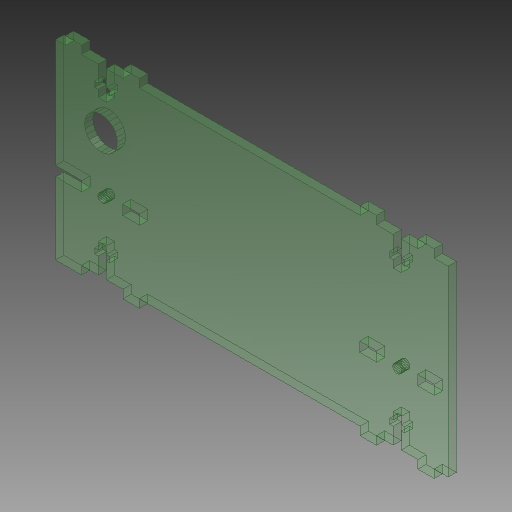
# Autodesk Inventor part: EE-Rear
Saved by Autodesk Inventor 2018 (Build 220112000, 112)
## iProperties
Created: 2016-07-27
Part Number: EE-Rear
Material: Polycarbonate, Green
Document SubType Name: Modeling
Designer: User
Density: 1.2 g/cm^3
Appearance: Polycarbonate - Clear(2)
Author: User
Autodesk Inventor part; units mm, degrees
ref_plane "YZ Plane" through (0, 0, 0) normal (1, 0, 0) x (0, 1, 0)
ref_plane "XZ Plane" through (0, 0, 0) normal (0, 1, 0) x (-1, 0, 0)
ref_plane "XY Plane" through (0, 0, 0) normal (0, 0, 1) x (1, 0, 0)
sketch "Sketch1" plane through (0, 0, 0) normal (0, 0, 1) x (1, 0, 0)
  line L0 (169.4009, -79.2776) -> (169.3009, -79.2776)
  line L1 (169.3009, -79.2776) -> (169.3009, -76.2776)
  line L2 (169.3009, -76.2776) -> (163.3009, -76.2776)
  line L3 (163.3009, -76.2776) -> (163.3009, -79.2776)
  line L4 (163.3009, -79.2776) -> (157.2009, -79.2776)
  line L5 (157.2009, -79.2776) -> (157.2009, -85.2776)
  line L6 (157.2009, -85.2776) -> (158.4509, -85.2776)
  line L7 (158.4509, -85.2776) -> (158.4509, -87.2776)
  line L8 (158.4509, -87.2776) -> (157.2009, -87.2776)
  line L9 (157.2009, -87.2776) -> (157.2009, -89.9276)
  line L10 (157.2009, -89.9276) -> (154.2009, -89.9276)
  line L11 (154.2009, -89.9276) -> (154.2009, -87.2776)
  line L12 (154.2009, -87.2776) -> (152.9509, -87.2776)
  line L13 (152.9509, -87.2776) -> (152.9509, -85.2776)
  line L14 (152.9509, -85.2776) -> (154.2009, -85.2776)
  line L15 (154.2009, -85.2776) -> (154.2009, -79.2776)
  line L16 (154.2009, -79.2776) -> (148.1009, -79.2776)
  line L17 (148.1009, -79.2776) -> (148.1009, -76.2776)
  line L18 (148.1009, -76.2776) -> (142.1009, -76.2776)
  line L19 (142.1009, -76.2776) -> (142.1009, -79.2776)
  line L20 (142.1009, -79.2776) -> (142.0009, -79.2776)
  line L21 (142.0009, -79.2776) -> (61.1009, -79.2776)
  line L22 (61.1009, -79.2776) -> (61.1009, -76.2776)
  line L23 (61.1009, -76.2776) -> (55.1009, -76.2776)
  line L24 (55.1009, -76.2776) -> (55.1009, -79.2776)
  line L25 (55.1009, -79.2776) -> (49.0009, -79.2776)
  line L26 (49.0009, -79.2776) -> (49.0009, -85.2776)
  line L27 (49.0009, -85.2776) -> (50.2509, -85.2776)
  line L28 (50.2509, -85.2776) -> (50.2509, -87.2776)
  line L29 (50.2509, -87.2776) -> (49.0009, -87.2776)
  line L30 (49.0009, -87.2776) -> (49.0009, -89.9276)
  line L31 (49.0009, -89.9276) -> (46.0009, -89.9276)
  line L32 (46.0009, -89.9276) -> (46.0009, -87.2776)
  line L33 (46.0009, -87.2776) -> (44.7509, -87.2776)
  line L34 (44.7509, -87.2776) -> (44.7509, -85.2776)
  line L35 (44.7509, -85.2776) -> (46.0009, -85.2776)
  line L36 (46.0009, -85.2776) -> (46.0009, -79.2776)
  line L37 (46.0009, -79.2776) -> (39.9009, -79.2776)
  line L38 (39.9009, -79.2776) -> (39.9009, -76.2776)
  line L39 (39.9009, -76.2776) -> (34.0009, -76.2776)
  line L40 (34.0009, -76.2776) -> (34.0009, -79.2776)
  line L41 (34.0009, -79.2776) -> (30.4009, -79.2776)
  line L42 (30.4009, -79.2776) -> (30.4009, -119.2776)
  line L43 (30.4009, -119.2776) -> (40.0009, -119.2776)
  line L44 (40.0009, -119.2776) -> (40.0009, -122.8776)
  line L45 (40.0009, -122.8776) -> (30.4009, -122.8776)
  line L46 (30.4009, -122.8776) -> (30.4009, -149.3251)
  line L47 (30.4009, -149.3251) -> (39.901, -149.3251)
  line L48 (39.901, -149.3251) -> (39.901, -146.2776)
  line L49 (39.901, -146.2776) -> (46.0009, -146.2776)
  line L50 (46.0009, -146.2776) -> (46.0009, -140.2776)
  line L51 (46.0009, -140.2776) -> (44.751, -140.2776)
  line L52 (44.751, -140.2776) -> (44.751, -138.2776)
  line L53 (44.751, -138.2776) -> (46.0009, -138.2776)
  line L54 (46.0009, -138.2776) -> (46.0009, -135.6276)
  line L55 (46.0009, -135.6276) -> (49.001, -135.6276)
  line L56 (49.001, -135.6276) -> (49.001, -138.2776)
  line L57 (49.001, -138.2776) -> (50.251, -138.2776)
  line L58 (50.251, -138.2776) -> (50.251, -140.2776)
  line L59 (50.251, -140.2776) -> (49.001, -140.2776)
  line L60 (49.001, -140.2776) -> (49.001, -146.2776)
  line L61 (49.001, -146.2776) -> (55.101, -146.2776)
  line L62 (55.101, -146.2776) -> (55.101, -149.3251)
  line L63 (55.101, -149.3251) -> (61.1009, -149.3251)
  line L64 (61.1009, -149.3251) -> (61.1009, -146.2776)
  line L65 (61.1009, -146.2776) -> (61.2009, -146.2776)
  line L66 (61.2009, -146.2776) -> (142.1009, -146.2776)
  line L67 (142.1009, -146.2776) -> (142.1009, -149.3251)
  line L68 (142.1009, -149.3251) -> (148.1009, -149.3251)
  line L69 (148.1009, -149.3251) -> (148.1009, -146.2776)
  line L70 (148.1009, -146.2776) -> (154.201, -146.2776)
  line L71 (154.201, -146.2776) -> (154.201, -140.2776)
  line L72 (154.201, -140.2776) -> (152.9509, -140.2776)
  line L73 (152.9509, -140.2776) -> (152.9509, -138.2776)
  line L74 (152.9509, -138.2776) -> (154.201, -138.2776)
  line L75 (154.201, -138.2776) -> (154.201, -135.6276)
  line L76 (154.201, -135.6276) -> (157.201, -135.6276)
  line L77 (157.201, -135.6276) -> (157.201, -138.2776)
  line L78 (157.201, -138.2776) -> (158.4509, -138.2776)
  line L79 (158.4509, -138.2776) -> (158.4509, -140.2776)
  line L80 (158.4509, -140.2776) -> (157.201, -140.2776)
  line L81 (157.201, -140.2776) -> (157.201, -146.2776)
  line L82 (157.201, -146.2776) -> (163.3009, -146.2776)
  line L83 (163.3009, -146.2776) -> (163.3009, -149.3251)
  line L84 (163.3009, -149.3251) -> (169.3009, -149.3251)
  line L85 (169.3009, -149.3251) -> (169.3009, -146.2776)
  line L86 (169.3009, -146.2776) -> (169.4009, -146.2776)
  line L87 (169.4009, -146.2776) -> (174.4009, -146.2776)
  line L88 (174.4009, -146.2776) -> (174.4009, -79.2776)
  line L89 (174.4009, -79.2776) -> (169.4009, -79.2776)
  line L90 (52.823, -99.1247) -> (52.2237, -97.6776)
  line L91 (52.2237, -97.6776) -> (51.2701, -96.435)
  line L92 (51.2701, -96.435) -> (50.0275, -95.4815)
  line L93 (50.0275, -95.4815) -> (48.5804, -94.8821)
  line L94 (48.5804, -94.8821) -> (47.0275, -94.6776)
  line L95 (47.0275, -94.6776) -> (45.4746, -94.8821)
  line L96 (45.4746, -94.8821) -> (44.0275, -95.4815)
  line L97 (44.0275, -95.4815) -> (42.7849, -96.435)
  line L98 (42.7849, -96.435) -> (41.8314, -97.6776)
  line L99 (41.8314, -97.6776) -> (41.232, -99.1247)
  line L100 (41.232, -99.1247) -> (41.0275, -100.6776)
  line L101 (41.0275, -100.6776) -> (41.232, -102.2306)
  line L102 (41.232, -102.2306) -> (41.8314, -103.6777)
  line L103 (41.8314, -103.6777) -> (42.7849, -104.9203)
  line L104 (42.7849, -104.9203) -> (44.0275, -105.8738)
  line L105 (44.0275, -105.8738) -> (45.4746, -106.4732)
  line L106 (45.4746, -106.4732) -> (47.0275, -106.6776)
  line L107 (47.0275, -106.6776) -> (48.5804, -106.4732)
  line L108 (48.5804, -106.4732) -> (50.0275, -105.8738)
  line L109 (50.0275, -105.8738) -> (51.2701, -104.9203)
  line L110 (51.2701, -104.9203) -> (52.2237, -103.6777)
  line L111 (52.2237, -103.6777) -> (52.823, -102.2306)
  line L112 (52.823, -102.2306) -> (53.0275, -100.6776)
  line L113 (53.0275, -100.6776) -> (52.823, -99.1247)
  line L114 (49.0226, -120.6837) -> (48.8518, -120.3208)
  line L115 (48.8518, -120.3208) -> (48.5962, -120.0117)
  line L116 (48.5962, -120.0117) -> (48.2718, -119.776)
  line L117 (48.2718, -119.776) -> (47.8988, -119.6284)
  line L118 (47.8988, -119.6284) -> (47.5009, -119.5781)
  line L119 (47.5009, -119.5781) -> (47.103, -119.6284)
  line L120 (47.103, -119.6284) -> (46.7301, -119.776)
  line L121 (46.7301, -119.776) -> (46.4056, -120.0117)
  line L122 (46.4056, -120.0117) -> (46.15, -120.3208)
  line L123 (46.15, -120.3208) -> (45.9792, -120.6837)
  line L124 (45.9792, -120.6837) -> (45.9041, -121.0776)
  line L125 (45.9041, -121.0776) -> (45.9293, -121.4779)
  line L126 (45.9293, -121.4779) -> (46.0532, -121.8594)
  line L127 (46.0532, -121.8594) -> (46.2681, -122.198)
  line L128 (46.2681, -122.198) -> (46.5605, -122.4725)
  line L129 (46.5605, -122.4725) -> (46.9119, -122.6657)
  line L130 (46.9119, -122.6657) -> (47.3004, -122.7655)
  line L131 (47.3004, -122.7655) -> (47.7014, -122.7655)
  line L132 (47.7014, -122.7655) -> (48.09, -122.6657)
  line L133 (48.09, -122.6657) -> (48.4414, -122.4725)
  line L134 (48.4414, -122.4725) -> (48.7337, -122.198)
  line L135 (48.7337, -122.198) -> (48.9486, -121.8594)
  line L136 (48.9486, -121.8594) -> (49.0726, -121.4779)
  line L137 (49.0726, -121.4779) -> (49.0978, -121.0776)
  line L138 (49.0978, -121.0776) -> (49.0226, -120.6837)
  line L139 (142.0009, -119.2776) -> (142.0009, -122.8776)
  line L140 (142.0009, -122.8776) -> (148.2009, -122.8776)
  line L141 (148.2009, -122.8776) -> (148.2009, -119.2776)
  line L142 (148.2009, -119.2776) -> (142.0009, -119.2776)
  line L143 (157.2226, -120.6837) -> (157.0518, -120.3208)
  line L144 (157.0518, -120.3208) -> (156.7962, -120.0117)
  line L145 (156.7962, -120.0117) -> (156.4717, -119.776)
  line L146 (156.4717, -119.776) -> (156.0988, -119.6284)
  line L147 (156.0988, -119.6284) -> (155.7009, -119.5781)
  line L148 (155.7009, -119.5781) -> (155.303, -119.6284)
  line L149 (155.303, -119.6284) -> (154.9301, -119.776)
  line L150 (154.9301, -119.776) -> (154.6056, -120.0117)
  line L151 (154.6056, -120.0117) -> (154.35, -120.3208)
  line L152 (154.35, -120.3208) -> (154.1792, -120.6837)
  line L153 (154.1792, -120.6837) -> (154.1041, -121.0776)
  line L154 (154.1041, -121.0776) -> (154.1292, -121.4779)
  line L155 (154.1292, -121.4779) -> (154.2532, -121.8594)
  line L156 (154.2532, -121.8594) -> (154.4681, -122.198)
  line L157 (154.4681, -122.198) -> (154.7605, -122.4725)
  line L158 (154.7605, -122.4725) -> (155.1119, -122.6657)
  line L159 (155.1119, -122.6657) -> (155.5004, -122.7655)
  line L160 (155.5004, -122.7655) -> (155.9014, -122.7655)
  line L161 (155.9014, -122.7655) -> (156.2899, -122.6657)
  line L162 (156.2899, -122.6657) -> (156.6414, -122.4725)
  line L163 (156.6414, -122.4725) -> (156.9337, -122.198)
  line L164 (156.9337, -122.198) -> (157.1487, -121.8594)
  line L165 (157.1487, -121.8594) -> (157.2726, -121.4779)
  line L166 (157.2726, -121.4779) -> (157.2978, -121.0776)
  line L167 (157.2978, -121.0776) -> (157.2226, -120.6837)
  line L168 (163.2009, -119.2776) -> (163.2009, -122.8776)
  line L169 (163.2009, -122.8776) -> (169.4009, -122.8776)
  line L170 (169.4009, -122.8776) -> (169.4009, -119.2776)
  line L171 (169.4009, -119.2776) -> (163.2009, -119.2776)
  line L172 (55.0009, -119.2776) -> (55.0009, -122.8776)
  line L173 (55.0009, -122.8776) -> (61.2009, -122.8776)
  line L174 (61.2009, -122.8776) -> (61.2009, -119.2776)
  line L175 (61.2009, -119.2776) -> (55.0009, -119.2776)
  point P0 (0, 0)
  constraints: 352 end point
extrude "Extrusion1" add sketch "Sketch1" along normal blind 3
body "Solid1"
